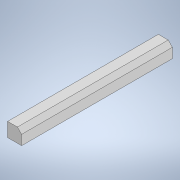
# Autodesk Inventor part: Shooter Base Cleat
Saved by Autodesk Inventor 2020 (Build 240168000, 168)
## iProperties
Created: 2020-02-01
Part Number: Shooter Base Cleat
Material: Generic
Document SubType Name: Modeling
Designer: JimAndVal
Density: 1 g/cm^3
Appearance: Default
Author: JimAndVal
Autodesk Inventor part; units mm, degrees
ref_plane "YZ Plane" through (0, 0, 0) normal (1, 0, 0) x (0, 1, 0)
ref_plane "XZ Plane" through (0, 0, 0) normal (0, 1, 0) x (-1, 0, 0)
ref_plane "XY Plane" through (0, 0, 0) normal (0, 0, 1) x (1, 0, 0)
sketch "Sketch1" plane through (0, 0, 0) normal (0, 0, 1) x (1, 0, 0)
  line L0 (12.7, -12.7) -> (-12.7, -12.7)
  line L1 (-12.7, -12.7) -> (-12.7, 12.7)
  line L2 (-12.7, 12.7) -> (5.08, 12.7)
  line L3 (12.7, 5.08) -> (12.7, -12.7)
  line L4 (12.7, -12.7) -> (-12.7, 12.7) construction
  line L5 (-12.7, -12.7) -> (12.7, 12.7) construction
  line L6 (5.08, 12.7) -> (12.7, 5.08)
  point P0 (0, 0)
  dimension "d0" = 25.4
  dimension "d1" = 25.4
  dimension "d2" = 7.62
  dimension "d3" = 7.62
  constraints: 14 end point, 2 midpoint, 2 parallel, 2 point on line, 1 horizontal, 1 perpendicular
  measures "d0" distance of L1.end L5.end
  measures "d1" distance of L0.end L1.end
  measures "d2" distance of L2.end L5.end
  measures "d3" distance of L3.start L5.end
extrude "Extrusion1" add sketch "Sketch1" along normal mid plane 273.05
equation "\"d3\" = d2"
body "Solid1"
